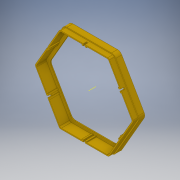
# Autodesk Inventor part: Cover v1
Saved by Autodesk Inventor 2019 (Build 230136000, 136)
## iProperties
Created: 2021-07-14
Part Number: Cover v1
Material: Generic
Document SubType Name: Modeling
Designer: Lix
Density: 1 g/cm^3
Appearance: Gold
d0: 175,000 mm
d1: 2,000 mm
d2: 0,00 deg
d15: 2,000 mm
d16: 2,000 mm
d17: 20,000 mm
d18: 0,00 deg
d19: 6,000 mm
d20: 7,000 mm
d21: 0,00 deg
d22: 10,000 mm
d23: 4,000 mm
d24: 10,000 mm
d25: 3,300 mm
d26: 6,500 mm
d27: 0,00 deg
d28: 4,000 mm
d29: 3,000 mm
d31: 0,00 deg
d32: 6,000 ul
d33: 360,00 deg
Author: Lix
Autodesk Inventor part; units mm, degrees
ref_plane "YZ Plane" through (0, 0, 0) normal (1, 0, 0) x (0, 1, 0)
ref_plane "XZ Plane" through (0, 0, 0) normal (0, 1, 0) x (-1, 0, 0)
ref_plane "XY Plane" through (0, 0, 0) normal (0, 0, 1) x (1, 0, 0)
sketch "Sketch1" plane through (0, 0, 0) normal (0, 0, 1) x (1, 0, 0)
  line L0 (50.5181, -87.5) -> (-50.5181, -87.5)
  line L1 (-50.5181, -87.5) -> (-101.0363, 0)
  line L2 (-101.0363, 0) -> (-50.5181, 87.5)
  line L3 (-50.5181, 87.5) -> (50.5181, 87.5)
  line L4 (50.5181, 87.5) -> (101.0363, 0)
  line L5 (101.0363, 0) -> (50.5181, -87.5)
  point P0 (0, 0)
  point P1 (0, 0)
  dimension "d0" = 175
  constraints: 12 end point, 1 coincident, 1 horizontal, 13 other
  measures "d0" distance between parallel lines of L4 L1
extrude "Extrusion1" add sketch "Sketch1" along normal blind 2
sketch "Sketch5" plane through (0, 0, 2) normal (0, 0, 1) x (1, 0, 0)
  line L0 (-50.5181, -87.5) -> (50.5181, -87.5) projected
  line L1 (50.5181, -87.5) -> (101.0363, 0) projected
  line L2 (101.0363, 0) -> (50.5181, 87.5) projected
  line L3 (50.5181, 87.5) -> (-50.5181, 87.5) projected
  line L4 (-50.5181, 87.5) -> (-101.0363, 0) projected
  line L5 (-101.0363, 0) -> (-50.5181, -87.5) projected
  line L6 (-98.7269, 0) -> (-49.3634, 85.5)
  line L7 (-49.3634, 85.5) -> (49.3634, 85.5)
  line L8 (49.3634, 85.5) -> (98.7269, 0)
  line L9 (98.7269, 0) -> (49.3634, -85.5)
  line L10 (49.3634, -85.5) -> (-49.3634, -85.5)
  line L11 (-49.3634, -85.5) -> (-98.7269, 0)
  line L12 (-96.4175, 0) -> (-48.2087, 83.5)
  line L13 (-48.2087, 83.5) -> (48.2087, 83.5)
  line L14 (48.2087, 83.5) -> (96.4175, 0)
  line L15 (96.4175, 0) -> (48.2087, -83.5)
  line L16 (48.2087, -83.5) -> (-48.2087, -83.5)
  line L17 (-48.2087, -83.5) -> (-96.4175, 0)
  point P0 (0, 0)
  dimension "d15" = 2
  dimension "d16" = 2
  constraints: 24 end point, 10 other
  measures "d15" distance between parallel lines of L4 L6
  measures "d16" distance between parallel lines of L11 L17
extrude "Extrusion5" add sketch "Sketch5" along normal blind 20 contours L6 L7 L8 L9 L10 L11
sketch "Sketch7" plane through (0, 0, 2) normal (0, 0, 1) x (1, 0, 0)
  line L0 (48.2087, 83.5) -> (-48.2087, 83.5) projected
  line L1 (-48.2087, 83.5) -> (-96.4175, 0) projected
  line L2 (-96.4175, 0) -> (-48.2087, -83.5) projected
  line L3 (-48.2087, -83.5) -> (48.2087, -83.5) projected
  line L4 (48.2087, -83.5) -> (96.4175, 0) projected
  line L5 (96.4175, 0) -> (48.2087, 83.5) projected
  line L6 (-44.7446, -77.5) -> (-89.4893, 0)
  line L7 (-89.4893, 0) -> (-44.7446, 77.5)
  line L8 (-44.7446, 77.5) -> (44.7446, 77.5)
  line L9 (44.7446, 77.5) -> (89.4893, 0)
  line L10 (89.4893, 0) -> (44.7446, -77.5)
  line L11 (44.7446, -77.5) -> (-44.7446, -77.5)
  point P0 (0, 0)
  dimension "d19" = 6
  constraints: 12 end point, 5 other
  measures "d19" distance between parallel lines of L2 L6
extrude "Extrusion6" cut sketch "Sketch7" against normal blind 7 contours L6 L7 L8 L9 L10 L11
fillet "Fillet1" radius 10 6 edges at (50.5181, 87.5, 1) (101.0363, 0, 1) (50.5181, -87.5, 1) (-50.5181, -87.5, 1) (-101.0363, 0, 1) (-50.5181, 87.5, 1)
fillet "Fillet1" radius 4 12 edges at (49.3634, -85.5, 12) (-48.2087, -83.5, 12) (-98.7269, 0, 12) (-49.3634, 85.5, 12) (49.3634, 85.5, 12) (98.7269, 0, 12) (48.2087, -83.5, 12) (96.4175, 0, 12) (-48.2087, 83.5, 12) (48.2087, 83.5, 12) (-49.3634, -85.5, 12) (-96.4175, 0, 12)
fillet "Fillet2" radius 10 6 edges at (44.7446, -77.5, 1) (89.4893, 0, 1) (44.7446, 77.5, 1) (-44.7446, 77.5, 1) (-89.4893, 0, 1) (-44.7446, -77.5, 1)
sketch "Sketch8" plane through (0, 0, 22) normal (0, 0, 1) x (1, 0, 0)
  line L0 (-1.65, 83.5) -> (1.65, 83.5)
  line L1 (1.65, 83.5) -> (1.65, 85.5)
  line L2 (1.65, 85.5) -> (-1.65, 85.5)
  line L3 (-1.65, 85.5) -> (-1.65, 83.5)
  line L4 (47.054, 85.5) -> (-47.054, 85.5) projected
  line L5 (-45.8993, 83.5) -> (45.8993, 83.5) projected
  point P0 (0, 0)
  point P1 (0, 85.5)
  point P2 (0, 85.5)
  point P3 (0, 0)
  dimension "d25" = 3.3
  constraints: 8 end point, 2 coincident, 2 collinear, 2 midpoint, 2 parallel, 1 horizontal, 1 perpendicular
  measures "d25" distance between parallel lines of L1 L3
extrude "Extrusion7" cut sketch "Sketch8" against normal blind 6.5
sketch "Sketch9" plane through (0, 0, 22) normal (0, 0, 1) x (1, 0, 0)
  line L0 (-4.65, 81.5) -> (-1.65, 81.5)
  line L1 (-1.65, 81.5) -> (-1.65, 85.5)
  line L2 (-1.65, 85.5) -> (-4.65, 85.5)
  line L3 (-4.65, 85.5) -> (-4.65, 81.5)
  line L4 (1.65, 83.5) -> (-1.65, 83.5) projected
  line L5 (1.65, 85.5) -> (1.65, 83.5) projected
  line L6 (-1.65, 85.5) -> (1.65, 85.5) projected
  line L7 (-1.65, 83.5) -> (-1.65, 85.5) projected
  line L8 (0, 83.5) -> (0, 81.6202) construction
  line L9 (-45.8993, 83.5) -> (-1.65, 83.5) projected
  line L10 (-1.65, 83.5) -> (-1.65, 85.5) projected
  line L11 (4.65, 81.5) -> (1.65, 81.5)
  line L12 (1.65, 81.5) -> (1.65, 85.5)
  line L13 (1.65, 85.5) -> (4.65, 85.5)
  line L14 (4.65, 85.5) -> (4.65, 81.5)
  line L15 (-1.65, 85.5) -> (-47.054, 85.5) projected
  point P0 (0, 0)
  dimension "d28" = 4
  dimension "d29" = 3
  constraints: 18 end point, 5 symmetric about line, 2 collinear, 2 parallel, 1 horizontal, 1 midpoint, 1 perpendicular, 1 vertical
  measures "d28" distance of L2.end L0.start
  measures "d29" distance of L1.end L2.end
extrude "Extrusion8" add sketch "Sketch9" against normal up to surface (20 mm away) contours L3 L9 L1 L0 | L3 L2 L1 L9 | L5 L13 L14 L11 L12
pattern_circular "Circular Pattern1" count 6 over 360 about axis through (0, 0, 0) along (0, 0, 1) of "Extrusion8", "Extrusion7"
sketch "Sketch11" plane through (0, 0, 2) normal (0, 0, 1) x (1, 0, 0)
  arc A0 (-44.7446, 87.5) -> (-53.4049, 82.5) centre (-44.7446, 77.5) ccw projected
  line L0 (-53.4049, 82.5) -> (-98.1495, 5) projected
  arc A1 (-98.1495, 5) -> (-98.1495, -5) centre (-89.4893, 0) ccw projected
  line L1 (-98.1495, -5) -> (-53.4049, -82.5) projected
  arc A2 (-53.4049, -82.5) -> (-44.7446, -87.5) centre (-44.7446, -77.5) ccw projected
  line L2 (-44.7446, -87.5) -> (44.7446, -87.5) projected
  arc A3 (44.7446, -87.5) -> (53.4049, -82.5) centre (44.7446, -77.5) ccw projected
  line L3 (53.4049, -82.5) -> (98.1495, -5) projected
  arc A4 (98.1495, -5) -> (98.1495, 5) centre (89.4893, 0) ccw projected
  line L4 (98.1495, 5) -> (53.4049, 82.5) projected
  arc A5 (53.4049, 82.5) -> (44.7446, 87.5) centre (44.7446, 77.5) ccw projected
  line L5 (44.7446, 87.5) -> (-44.7446, 87.5) projected
  line L6 (-47.054, 85.5) -> (47.054, 85.5) projected
  arc A6 (50.5181, 83.5) -> (47.054, 85.5) centre (47.054, 81.5) ccw projected
  line L7 (50.5181, 83.5) -> (97.5722, 2) projected
  arc A7 (97.5722, -2) -> (97.5722, 2) centre (94.1081, 0) ccw projected
  line L8 (97.5722, -2) -> (50.5181, -83.5) projected
  arc A8 (47.054, -85.5) -> (50.5181, -83.5) centre (47.054, -81.5) ccw projected
  line L9 (47.054, -85.5) -> (-47.054, -85.5) projected
  arc A9 (-50.5181, -83.5) -> (-47.054, -85.5) centre (-47.054, -81.5) ccw projected
  line L10 (-50.5181, -83.5) -> (-97.5722, -2) projected
  arc A10 (-97.5722, 2) -> (-97.5722, -2) centre (-94.1081, 0) ccw projected
  line L11 (-97.5722, 2) -> (-50.5181, 83.5) projected
  arc A11 (-47.054, 85.5) -> (-50.5181, 83.5) centre (-47.054, 81.5) ccw projected
  point P0 (0, 0)
extrude "Extrusion9" add sketch "Sketch11" along normal blind 10
body "Solid1"
